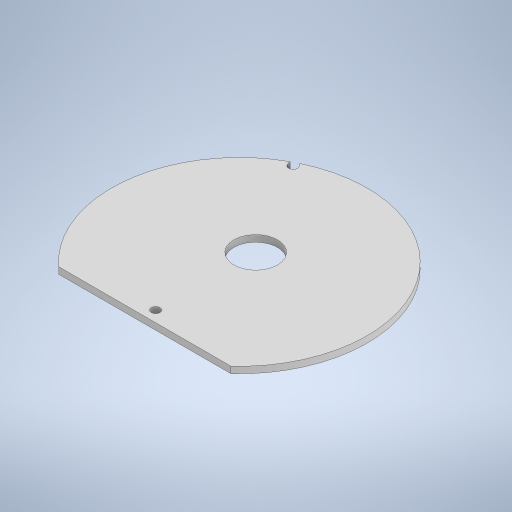
# Autodesk Inventor part: Cover
Saved by Autodesk Inventor 2024.2 (Build 282272000, 272)
## iProperties
Created: 2024-04-10
Part Number: Cover
Material: Generic
Document SubType Name: Modeling
Designer: Micha
Density: 1 g/cm^3
Appearance: Default
Author: Micha
Autodesk Inventor part; units mm, degrees
ref_plane "YZ Plane" through (0, 0, 0) normal (1, 0, 0) x (0, 1, 0)
ref_plane "XZ Plane" through (0, 0, 0) normal (0, 1, 0) x (-1, 0, 0)
ref_plane "XY Plane" through (0, 0, 0) normal (0, 0, 1) x (1, 0, 0)
sketch "Sketch1" plane through (0, 0, 0) normal (0, 1, 0) x (-1, 0, 0)
  arc A0 (-39.616, 43.7215) -> (39.616, 43.7215) centre (0, 0) ccw construction
  line L0 (39.616, 43.7215) -> (-39.616, 43.7215)
  arc A1 (-39.4614, 43.3215) -> (39.4614, 43.3215) centre (0, 0) ccw
  line L1 (-39.4614, 43.3215) -> (39.4614, 43.3215)
  circle A2 centre (0, -7.5) radius 10
  circle A3 centre (0, 38.3215) radius 2
  circle A4 centre (25.7608, -50.3979) radius 2
  line L2 (27.6746, -49.8171) -> (28.1531, -51.3942)
  line L3 (24.1691, -51.6089) -> (25.1671, -52.9205)
  dimension "d0" = 118
  dimension "d1" = 79.232
  dimension "d2" = 0.4
  dimension "d3" = 20
  dimension "d4" = 7.5
  dimension "d5" = 4
  dimension "d6" = 5
  dimension "d7" = 4
  constraints: 8 end point, 8 point on circle, 5 centre point, 3 tangent, 2 vertical alignment, 1 coincident, 1 equal length, 1 horizontal, 1 other
  measures "d0" diameter of A0
  measures "d1" distance of L0.start L0.end
  measures "d2" radial gap between concentric circles of A0 A1
  measures "d3" diameter of A2
  measures "d4" distance of point (0, 0) A2.centre
  measures "d5" diameter of A3
  measures "d6" distance from line of L1 A3.centre
  measures "d7" diameter of A4
extrude "Extrusion1" add sketch "Sketch1" along normal blind 3 contours L1 A1 L2 A4 L3
body "Solid1"
